seal_wall_holder (Autodesk Fusion 360 design; units mm, degrees)
Autodesk Fusion 360 part; units mm, degrees
sketch "Sketch1" plane through (0, 0, 0) normal (0, 0, 1) x (1, 0, 0)
  line L0 (0, 0) -> (-50, 0)
  line L1 (-50, 0) -> (-50, 115)
  line L2 (-50, 115) -> (0, 115)
  line L3 (0, 115) -> (0, 0)
  line L4 (-50, 115) -> (0, 139.3866)
  line L5 (0, 139.3866) -> (0, 115)
  line L6 (-50, 115) -> (-51.7535, 118.5952)
  line L7 (-51.7535, 118.5952) -> (-1.7535, 142.9818)
  line L8 (-1.7535, 142.9818) -> (0, 139.3866)
  spline S0 degree 5 poles (-50, 115) (-49.1286, 114.1162) (-47.4651, 112.3243) (-45.2074, 109.5639) (-42.6804, 105.7358) (-40.3787, 100.6888) (-38.9992, 95.3602) (-38.5993, 89.7323) (-39.1781, 83.8055) (-40.6677, 77.6006) (-42.9855, 71.1426) (-45.4417, 65.7923) (-47.6, 61.6831) (-49.177, 58.9014) (-50, 57.5) knots 0 0 0 0 0 0 0.1 0.2 0.3 0.4 0.5 0.6 0.7 0.8 0.9 1 1 1 1 1 1
  spline S1 degree 5 poles (0, 139.3866) (-0.8361, 137.4921) (-2.4376, 133.7247) (-4.6279, 128.1387) (-7.1171, 120.8232) (-9.4593, 111.9151) (-10.9559, 103.2668) (-11.5257, 94.9031) (-11.1043, 86.8438) (-9.6988, 79.0869) (-7.3699, 71.6136) (-4.822, 65.8453) (-2.5494, 61.6301) (-0.8762, 58.8686) (0, 57.5) knots 0 0 0 0 0 0 0.1 0.2 0.3 0.4 0.5 0.6 0.7 0.8 0.9 1 1 1 1 1 1
  point P0 (-38.8957, 92.1099)
  point P1 (-11.243, 92.1099)
  dimension "d1" = 50
  dimension "d2" = 115
  dimension "d3" = 26
  dimension "d4" = 4
  constraint horizontal L0
  constraint vertical L1
  constraint horizontal L2
  constraint vertical L3
  constraint coincident L0.start L3.end
  constraint collinear L3 L5
  constraint perpendicular L4 L6
  constraint perpendicular L6 L7
  constraint perpendicular L7 L8
  constraint midpoint L1 S0.end
  constraint midpoint L3 S1.end
  measures "d1" distance of L0.start L0.end
  measures "d2" distance of L0.start L2.end
  measures "d3" angle of L2 L4
  measures "d4" distance of L4 L7
extrude "Extrude1" add sketch "Sketch1" along normal blind 4 contours L0 L1 L2 L3 S0 S1 | L2 L4 S1 | L4 L6 L7 L8
extrude "Extrude2" add sketch "Sketch1" along normal blind 35 contours L4 L6 L7 L8
fillet "Fillet1" radius 20 2 edges at (-50.8767, 116.7976, 35) (-0.8767, 141.1842, 35)
fillet "Fillet2" radius 25 2 edges at (-50, 0, 2) (0, 0, 2)
fillet "Fillet3" radius 147.5 2 edges at (0, 57.5, 2) (-50, 57.5, 2)
sketch "Sketch2" plane through (-54.9191, 112.6008, 0) normal (0.438371, -0.898794, 0) x (0.898794, 0.438371, 0)
  arc A0 (61.1031, 15) -> (41.1031, 35) centre (41.1031, 15) ccw
  line L0 (41.1031, 35) -> (25.473, 35)
  arc A1 (25.473, 35) -> (5.473, 15) centre (25.473, 15) ccw
  line L1 (5.473, 15) -> (5.473, 4)
  line L2 (5.473, 4) -> (61.1031, 4)
  line L3 (61.1031, 4) -> (61.1031, 15)
  circle A2 centre (32.4556, 24.4508) radius 1.5
  dimension "d15" = 3
  measures "d15" diameter of A2
extrude "Extrude3" cut sketch "Sketch2" against normal blind 20 contours A2
